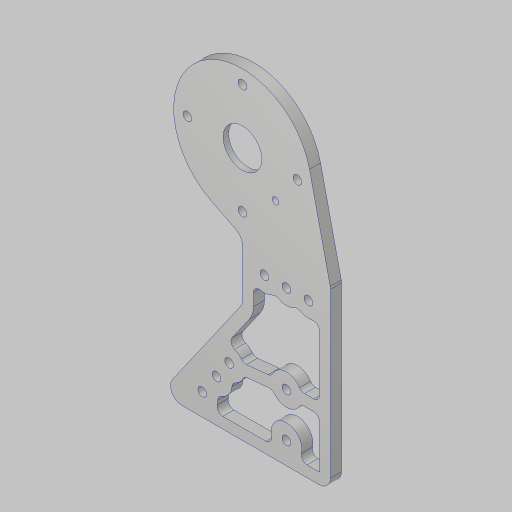
# Autodesk Inventor part: CL7-010
Saved by Autodesk Inventor 2023.5 (Build 275446000, 446)
## iProperties
Created: 2025-03-18
Part Number: CL7-010
Material: Aluminum 6061
Document SubType Name: Modeling
Designer: slick
Density: 2.7 g/cm^3
Appearance: Aluminum - Flat
Author: slick
Autodesk Inventor part; units mm, degrees
ref_plane "YZ Plane" through (0, 0, 0) normal (1, 0, 0) x (0, 1, 0)
ref_plane "XZ Plane" through (0, 0, 0) normal (0, 1, 0) x (-1, 0, 0)
ref_plane "XY Plane" through (0, 0, 0) normal (0, 0, 1) x (1, 0, 0)
sketch "Sketch1" plane through (0, 0, 0) normal (0, 0, 1) x (1, 0, 0)
  line L0 (0, 0) -> (50.8, 0) construction
  line L1 (50.8, 0) -> (50.8, 387.35) construction
  line L2 (50.8, 387.35) -> (0, 387.35) construction
  line L3 (0, 387.35) -> (0, 0) construction
  line L4 (20.8065, 339.141) -> (-226.8638, -14.5688) construction
  line L5 (-226.8638, -14.5688) -> (-247.6703, 0) construction
  line L6 (-247.6703, 0) -> (0, 353.7099) construction
  line L7 (0, 353.7099) -> (20.8065, 339.141) construction
  line L8 (-247.6703, 0) -> (-216.6626, 0) construction
  line L9 (0, 353.7099) -> (0, 309.4263) construction
  dimension "d0" = 50.8
  dimension "d1" = 387.35
  dimension "d2" = 25.4
  dimension "d3" = 431.8
  dimension "d5" = 55
  constraints: 20 end point, 4 parallel, 2 horizontal, 2 perpendicular, 2 point on line, 1 horizontal alignment, 1 vertical, 1 vertical alignment
  measures "d0" distance of L2.end L1.end
  measures "d1" distance of L1.end L0.end
  measures "d2" distance of L4.end L5.end
  measures "d3" distance of L5.end L6.end
  measures "d5" angle of L7 L3
sketch "Sketch2" plane through (0, 0, 0) normal (0, 0, 1) x (1, 0, 0)
  line L0 (0, 0) -> (50.8, 0) construction
  line L1 (50.8, 0) -> (50.8, 387.35) construction
  line L2 (50.8, 387.35) -> (0, 387.35) construction
  line L3 (0, 387.35) -> (0, 0) construction
  line L4 (20.8065, 339.141) -> (-226.8638, -14.5688) construction
  line L5 (-226.8638, -14.5688) -> (-247.6703, 0) construction
  line L6 (-247.6703, 0) -> (0, 353.7099) construction
  line L7 (0, 353.7099) -> (20.8065, 339.141) construction
  line L8 (-247.6703, 0) -> (-216.6626, 0) construction
  line L9 (0, 353.7099) -> (0, 309.4263) construction
  circle A0 centre (0, 431.8) radius 11.176
  circle A1 centre (0, 431.8) radius 23.8125 construction
  circle A2 centre (0, 431.8) radius 39.6875 construction
  line L10 (-47.586, 285.75) -> (0, 353.7099)
  line L11 (0, 387.35) -> (0, 353.7099)
  line L12 (0, 387.35) -> (-17.8729, 396.3647)
  line L13 (50.8, 387.35) -> (50.8, 285.75)
  line L14 (50.8, 285.75) -> (-47.586, 285.75)
  arc A3 (38.7009, 440.5943) -> (-17.8729, 396.3647) centre (0, 431.8) ccw
  line L15 (12.7, 374.65) -> (38.1, 374.65) construction
  line L16 (10.4032, 346.4254) -> (-237.2671, -7.2844) construction
  line L17 (50.8, 387.35) -> (38.7009, 440.5943)
  point P0 (25.4, 0)
  point P1 (-7.667, 320.6184)
  point P2 (-14.9514, 310.2152)
  point P3 (-23.1895, 298.45)
  point P4 (25.4, 374.65)
  point P5 (25.4, 374.65)
  point P6 (25.4, 387.35)
  dimension "d6" = 22.352
  dimension "d7" = 47.625
  dimension "d8" = 15.875
  dimension "d11" = 431.8
  dimension "d12" = 101.6
  dimension "d13" = 25.4
  dimension "d14" = 12.7
  dimension "d15" = 12.7
  dimension "d16" = 14.3627
  dimension "d17" = 12.7
  dimension "d52" = 50.8
  constraints: 16 end point, 5 midpoint, 5 point on line, 4 centre point, 4 point on circle, 3 coincident, 2 perpendicular, 2 tangent, 1 collinear, 1 horizontal, 1 vertical alignment
  measures "d6" diameter of A0
  measures "d7" diameter of A1
  measures "d8" radial gap between concentric circles of A1 A2
  measures "d11" distance from line of L0 A0.centre
  measures "d12" distance between parallel lines of L2 L14
  measures "d13" distance of L15.start L15.end
  measures "d14" distance between parallel lines of L2 L15
  measures "d15" distance of point (-14.951, 310.215) point (-7.667, 320.618)
  measures "d16" distance of point (-14.951, 310.215) point (-23.19, 298.45)
  measures "d17" distance from line of L14 point (-23.19, 298.45)
  measures "d52" distance from line of L1 A0.centre
extrude "Extrusion1" add sketch "Sketch2" along normal blind 6.35
hole "Hole1" at (0, 0, 0) at (50.8, 0, 0) at (-226.8638, -14.5688, 0) at (-247.6703, 0, 0) at (-216.6626, 0, 0) at (-7.667, 320.6184, 0) at (-14.9514, 310.2152, 0) at (-23.1895, 298.45, 0) at (12.7, 374.65, 0) at (25.4, 374.65, 0) at (38.1, 374.65, 0) direction (0, 0, 1) diameter 5.1054 end through all clearance for "Flat Head Machine Screw (82)" size "#10" standard "Ansi Unified Screw Threads"
fillet "Fillet1" radius 6.604 5 edges at (0, 353.7099, 3.175) (-47.586, 285.75, 3.175) (50.8, 285.75, 3.175) (0, 387.35, 3.175) (50.8, 387.35, 3.175)
sketch "Sketch3" plane through (0, 0, 0) normal (0, 0, -1) x (-1, 0, 0)
  arc A0 (-50.8, 292.354) -> (-44.196, 285.75) centre (-44.196, 292.354) ccw construction
  line L0 (34.8998, 285.75) -> (-44.196, 285.75) construction
  arc A1 (34.8998, 285.75) -> (40.3095, 296.1419) centre (34.8998, 292.354) ccw construction
  line L1 (1.1943, 352.0042) -> (40.3095, 296.1419) construction
  arc A2 (0, 355.7921) -> (1.1943, 352.0042) centre (6.604, 355.7921) ccw construction
  line L2 (0, 383.2845) -> (0, 355.7921) construction
  line L3 (17.8729, 396.3647) -> (3.63, 389.1809) construction
  arc A3 (17.8729, 396.3647) -> (-38.7009, 440.5943) centre (0, 431.8) ccw construction
  line L4 (-50.8, 292.354) -> (-50.8, 386.6091) construction
  circle A4 centre (-25.4, 374.65) radius 2.5527 construction
  circle A5 centre (23.1895, 298.45) radius 2.5527 construction
  circle A6 centre (7.667, 320.6184) radius 2.5527 construction
  circle A7 centre (14.9514, 310.2152) radius 2.5527 construction
  circle A8 centre (-12.7, 374.65) radius 2.5527 construction
  circle A9 centre (-38.1, 374.65) radius 2.5527 construction
  circle A10 centre (0, 431.8) radius 11.176 construction
  circle A11 centre (0, 431.8) radius 23.8125
  circle A12 centre (0, 431.8) radius 11.176 construction
  circle A13 centre (0, 431.8) radius 31.75 construction
  line L5 (-50.6358, 388.0725) -> (-38.7009, 440.5943) projected
  arc A14 (-50.6358, 388.0725) -> (-50.8, 386.6091) centre (-44.196, 386.6091) ccw projected
  arc A15 (3.63, 389.1809) -> (0, 383.2845) centre (6.604, 383.2845) ccw projected
  point P0 (0, 0)
  point P1 (0, 463.55)
  point P2 (-31.75, 431.8)
  point P3 (0, 400.05)
  point P4 (31.75, 431.8)
  dimension "d29" = 63.5
  dimension "d28" = 47.625
  dimension "d32" = 360
  constraints: 2 coincident, 2 vertical alignment, 1 centre point, 7 other
  measures "d28" diameter of A11
extrude "Extrusion2" cut sketch "Sketch3" against normal blind 3.175
hole "Hole2" at (0, 463.55, 0) at (31.75, 431.8, 0) at (0, 400.05, 0) at (-31.75, 431.8, 0) direction (0, 0, 1) diameter 5.1054 end through all clearance for "Flat Head Machine Screw (82)" size "#10" standard "Ansi Unified Screw Threads"
sketch "Sketch4" plane through (0, 0, 6.35) normal (0, 0, 1) x (1, 0, 0)
  line L0 (0, 0) -> (50.8, 0) construction
  line L1 (-34.8998, 285.75) -> (44.196, 285.75) construction
  point P0 (25.4, 323.85)
  point P1 (25.4, 298.45)
  point P2 (25.4, 0)
  dimension "d43" = 25.4
  dimension "d44" = 12.7
  constraints: 2 vertical alignment, 1 midpoint
  measures "d43" distance of point (25.4, 323.85) point (25.4, 298.45)
  measures "d44" distance from line of L1 point (25.4, 298.45)
hole "Hole3" at (25.4, 323.85, 6.35) at (25.4, 298.45, 6.35) direction (0, 0, -1) diameter 5.1054 end through all clearance for "Flat Head Machine Screw (82)" size "#10" standard "Ansi Unified Screw Threads"
sketch "Sketch5" plane through (0, 0, 6.35) normal (0, 0, 1) x (1, 0, 0)
  circle A0 centre (25.4, 323.85) radius 2.5527 construction
  circle A1 centre (25.4, 298.45) radius 2.5527 construction
  circle A2 centre (0, 400.05) radius 2.5527 construction
  circle A3 centre (0, 463.55) radius 2.5527 construction
  circle A4 centre (31.75, 431.8) radius 2.5527 construction
  circle A5 centre (-31.75, 431.8) radius 2.5527 construction
  circle A6 centre (0, 431.8) radius 11.176 construction
  arc A7 (50.8, 386.6091) -> (50.6358, 388.0725) centre (44.196, 386.6091) ccw construction
  line L0 (50.6358, 388.0725) -> (38.7009, 440.5943) construction
  arc A8 (38.7009, 440.5943) -> (-17.8729, 396.3647) centre (0, 431.8) ccw construction
  line L1 (-17.8729, 396.3647) -> (-3.63, 389.1809) construction
  arc A9 (0, 383.2845) -> (-3.63, 389.1809) centre (-6.604, 383.2845) ccw construction
  line L2 (0, 383.2845) -> (0, 355.7921) construction
  arc A10 (-1.1943, 352.0042) -> (0, 355.7921) centre (-6.604, 355.7921) ccw construction
  line L3 (-1.1943, 352.0042) -> (-40.3095, 296.1419) construction
  arc A11 (-40.3095, 296.1419) -> (-34.8998, 285.75) centre (-34.8998, 292.354) ccw construction
  line L4 (-34.8998, 285.75) -> (44.196, 285.75) construction
  arc A12 (44.196, 285.75) -> (50.8, 292.354) centre (44.196, 292.354) ccw construction
  line L5 (50.8, 292.354) -> (50.8, 386.6091) construction
  circle A13 centre (38.1, 374.65) radius 2.5527 construction
  circle A14 centre (12.7, 374.65) radius 2.5527 construction
  circle A15 centre (-14.9514, 310.2152) radius 2.5527 construction
  circle A16 centre (-7.667, 320.6184) radius 2.5527 construction
  circle A17 centre (-23.1895, 298.45) radius 2.5527 construction
  circle A18 centre (25.4, 374.65) radius 2.5527 construction
  line L6 (6.35, 355.7921) -> (6.35, 383.2845) construction
  arc A19 (6.35, 383.2845) -> (-0.7703, 394.8505) centre (-6.604, 383.2845) ccw construction
  line L7 (-0.7703, 394.8505) -> (-15.0132, 402.0344) construction
  arc A20 (32.5087, 439.1872) -> (-15.0132, 402.0344) centre (0, 431.8) ccw construction
  line L8 (32.5087, 439.1872) -> (44.4437, 386.6654) construction
  arc A21 (44.45, 386.6091) -> (44.4437, 386.6654) centre (44.196, 386.6091) ccw construction
  line L9 (44.45, 386.6091) -> (44.45, 292.354) construction
  arc A22 (44.196, 292.1) -> (44.45, 292.354) centre (44.196, 292.354) ccw construction
  line L10 (44.196, 292.1) -> (-34.8998, 292.1) construction
  arc A23 (-35.1079, 292.4997) -> (-34.8998, 292.1) centre (-34.8998, 292.354) ccw construction
  line L11 (-35.1079, 292.4997) -> (4.0073, 348.362) construction
  arc A24 (4.0073, 348.362) -> (6.35, 355.7921) centre (-6.604, 355.7921) ccw construction
  circle A25 centre (25.4, 323.85) radius 8.9027 construction
  circle A26 centre (12.7, 374.65) radius 8.9027 construction
  circle A27 centre (25.4, 374.65) radius 8.9027 construction
  circle A28 centre (38.1, 374.65) radius 8.9027 construction
  circle A29 centre (-7.667, 320.6184) radius 2.5527 construction
  circle A30 centre (-7.667, 320.6184) radius 8.9027 construction
  line L12 (-7.667, 320.6184) -> (25.4, 323.85) construction
  line L13 (25.4, 323.85) -> (44.45, 323.85) construction
  arc A31 (6.35, 368.4102) -> (19.05, 368.4102) centre (12.7, 374.65) ccw
  arc A32 (19.05, 368.4102) -> (31.75, 368.4102) centre (25.4, 374.65) ccw
  arc A33 (31.75, 368.4102) -> (44.45, 368.4102) centre (38.1, 374.65) ccw
  arc A34 (-1.1943, 352.0042) -> (0, 355.7921) centre (-6.604, 355.7921) ccw construction
  arc A35 (4.0073, 348.362) -> (6.35, 355.7921) centre (-6.604, 355.7921) ccw
  line L14 (6.35, 368.4102) -> (6.35, 355.7921)
  line L15 (44.45, 323.85) -> (44.45, 368.4102)
  line L16 (4.0073, 348.362) -> (-9.2896, 329.372)
  circle A36 centre (0, 431.8) radius 33.3375 construction
  circle A37 centre (0, 400.05) radius 8.9027 construction
  circle A38 centre (31.75, 431.8) radius 2.5527 construction
  circle A39 centre (31.75, 431.8) radius 8.9027 construction
  circle A40 centre (0, 431.8) radius 36.5125 construction
  arc A41 (8.0168, 396.1785) -> (35.6215, 423.7832) centre (0, 431.8) ccw
  arc A42 (3.2058, 391.7445) -> (8.0168, 396.1785) centre (0, 400.05) ccw
  arc A43 (35.6215, 423.7832) -> (35.9688, 423.9604) centre (31.75, 431.8) ccw
  arc A44 (44.45, 386.6091) -> (44.4437, 386.6654) centre (44.196, 386.6091) ccw
  arc A45 (6.35, 383.2845) -> (3.2058, 391.7445) centre (-6.604, 383.2845) ccw
  arc A46 (19.05, 380.8898) -> (6.35, 380.8898) centre (12.7, 374.65) ccw
  arc A47 (31.75, 380.8898) -> (19.05, 380.8898) centre (25.4, 374.65) ccw
  arc A48 (44.45, 380.8898) -> (31.75, 380.8898) centre (38.1, 374.65) ccw
  line L17 (6.35, 383.2845) -> (6.35, 380.8898)
  line L18 (44.45, 380.8898) -> (44.45, 386.6091)
  line L19 (44.4437, 386.6654) -> (35.9688, 423.9604)
  circle A49 centre (-23.1895, 298.45) radius 8.9027 construction
  circle A50 centre (25.4, 298.45) radius 8.9027 construction
  circle A51 centre (-14.9514, 310.2152) radius 8.9027 construction
  line L20 (-7.9758, 323.7784) -> (25.2452, 327.025) construction
  line L21 (25.2452, 327.025) -> (44.45, 327.025) construction
  line L22 (-7.3582, 317.4585) -> (25.5548, 320.675) construction
  line L23 (25.5548, 320.675) -> (44.45, 320.675) construction
  line L24 (0.302, 324.5874) -> (16.8133, 326.201)
  line L25 (33.7173, 327.025) -> (44.45, 327.025)
  line L26 (44.45, 320.675) -> (33.7173, 320.675)
  line L27 (17.431, 319.8811) -> (0.9197, 318.2675)
  line L28 (44.45, 320.675) -> (44.45, 292.354)
  line L29 (44.196, 292.1) -> (31.6398, 292.1)
  line L30 (19.1602, 292.1) -> (-16.9497, 292.1)
  arc A52 (-16.9497, 292.1) -> (-14.7603, 301.3146) centre (-23.1895, 298.45) ccw
  arc A53 (-14.7603, 301.3146) -> (-6.1979, 311.8378) centre (-14.9514, 310.2152) ccw
  arc A54 (-6.1979, 311.8378) -> (0.9197, 318.2675) centre (-7.667, 320.6184) ccw
  arc A55 (17.431, 319.8811) -> (33.7173, 320.675) centre (25.4, 323.85) ccw
  arc A56 (33.7173, 327.025) -> (16.8133, 326.201) centre (25.4, 323.85) ccw
  arc A57 (31.6398, 292.1) -> (19.1602, 292.1) centre (25.4, 298.45) ccw
  arc A58 (44.196, 292.1) -> (44.45, 292.354) centre (44.196, 292.354) ccw
  arc A59 (0.302, 324.5874) -> (-9.2896, 329.372) centre (-7.667, 320.6184) ccw
  point P0 (0, 0)
  point P1 (1.1935, 321.4844)
  point P2 (34.3027, 323.85)
  point P3 (16.5395, 322.9841)
  point P4 (44.45, 386.6091)
  dimension "d53" = 6.35
  dimension "d54" = 6.35
  dimension "d55" = 3.175
  dimension "d60" = 3.175
  dimension "d61" = 3.175
  constraints: 88 point on circle, 50 end point, 38 centre point, 30 coincident, 21 point on line, 11 equal radius, 4 collinear, 1 perpendicular, 13 other
  measures "d53" distance between parallel lines of L2 L6
  measures "d54" radial gap between concentric circles of A0 A25
  measures "d55" radial gap between concentric circles of A36 A40
  measures "d60" distance between parallel lines of L12 L20
  measures "d61" distance between parallel lines of L12 L22
extrude "Extrusion3" cut sketch "Sketch5" against normal through all contours A31 A32 A33 L15 L25 A56 L24 A59 L16 A35 L14 | L28 A58 L29 A57 L30 A52 A53 A54 L27 A55 L26
fillet "Fillet2" radius 3.302 18 edges at (-16.9497, 292.1, 3.175) (19.1602, 292.1, 3.175) (31.6398, 292.1, 3.175) (44.45, 320.675, 3.175) (33.7173, 320.675, 3.175) (17.431, 319.8811, 3.175) (0.9197, 318.2675, 3.175) (-6.1979, 311.8378, 3.175) (-14.7603, 301.3146, 3.175) (16.8133, 326.201, 3.175) (33.7173, 327.025, 3.175) (44.45, 327.025, 3.175) (44.45, 368.4102, 3.175) (31.75, 368.4102, 3.175) (19.05, 368.4102, 3.175) (6.35, 368.4102, 3.175) (-9.2896, 329.372, 3.175) (0.302, 324.5874, 3.175)
sketch "Sketch6" plane through (0, 0, 6.35) normal (0, 0, 1) x (1, 0, 0)
  line L0 (35.7442, 320.675) -> (41.148, 320.675) construction
  arc A0 (44.45, 317.373) -> (41.148, 320.675) centre (41.148, 317.373) ccw construction
  line L1 (44.45, 317.373) -> (44.45, 292.354) construction
  arc A1 (44.196, 292.1) -> (44.45, 292.354) centre (44.196, 292.354) ccw construction
  line L2 (44.196, 292.1) -> (37.218, 292.1) construction
  arc A2 (34.0206, 296.2266) -> (37.218, 292.1) centre (37.218, 295.402) ccw construction
  arc A3 (34.0206, 296.2266) -> (16.7794, 296.2266) centre (25.4, 298.45) ccw construction
  arc A4 (13.582, 292.1) -> (16.7794, 296.2266) centre (13.582, 295.402) ccw construction
  line L3 (13.582, 292.1) -> (-11.3716, 292.1) construction
  arc A5 (-14.5689, 296.2266) -> (-11.3716, 292.1) centre (-11.3716, 295.402) ccw construction
  arc A6 (-14.5689, 296.2266) -> (-14.2883, 298.6122) centre (-23.1895, 298.45) ccw construction
  arc A7 (-12.0595, 301.7953) -> (-14.2883, 298.6122) centre (-10.9869, 298.6724) ccw construction
  arc A8 (-12.0595, 301.7953) -> (-6.0668, 309.6487) centre (-14.9514, 310.2152) ccw construction
  arc A9 (-4.096, 312.4633) -> (-6.0668, 309.6487) centre (-2.7715, 309.4386) ccw construction
  arc A10 (-4.096, 312.4633) -> (0.3023, 316.6501) centre (-7.667, 320.6184) ccw construction
  arc A11 (2.937, 318.4646) -> (0.3023, 316.6501) centre (3.2581, 315.1783) ccw construction
  line L4 (2.937, 318.4646) -> (15.4136, 319.6839) construction
  arc A12 (18.3497, 318.4138) -> (15.4136, 319.6839) centre (15.7348, 316.3976) ccw construction
  arc A13 (18.3497, 318.4138) -> (32.9456, 319.1254) centre (25.4, 323.85) ccw construction
  arc A14 (35.7442, 320.675) -> (32.9456, 319.1254) centre (35.7442, 317.373) ccw construction
  arc A15 (10.4766, 366.0294) -> (17.332, 367.0472) centre (12.7, 374.65) ccw construction
  arc A16 (20.768, 367.0472) -> (17.332, 367.0472) centre (19.05, 364.2273) ccw construction
  arc A17 (20.768, 367.0472) -> (30.032, 367.0472) centre (25.4, 374.65) ccw construction
  arc A18 (33.468, 367.0472) -> (30.032, 367.0472) centre (31.75, 364.2273) ccw construction
  arc A19 (33.468, 367.0472) -> (40.3234, 366.0294) centre (38.1, 374.65) ccw construction
  arc A20 (44.45, 362.832) -> (40.3234, 366.0294) centre (41.148, 362.832) ccw construction
  line L5 (44.45, 362.832) -> (44.45, 330.327) construction
  arc A21 (41.148, 327.025) -> (44.45, 330.327) centre (41.148, 330.327) ccw construction
  line L6 (41.148, 327.025) -> (35.7442, 327.025) construction
  arc A22 (32.9456, 328.5746) -> (35.7442, 327.025) centre (35.7442, 330.327) ccw construction
  arc A23 (32.9456, 328.5746) -> (17.4307, 327.8183) centre (25.4, 323.85) ccw construction
  arc A24 (14.796, 326.0038) -> (17.4307, 327.8183) centre (14.4748, 329.2902) ccw construction
  line L7 (14.796, 326.0038) -> (2.3194, 324.7845) construction
  arc A25 (-0.6167, 326.0546) -> (2.3194, 324.7845) centre (1.9982, 328.0709) ccw construction
  arc A26 (-0.6167, 326.0546) -> (-4.5437, 328.9553) centre (-7.667, 320.6184) ccw construction
  arc A27 (-6.0901, 333.9414) -> (-4.5437, 328.9553) centre (-3.3853, 332.0474) ccw construction
  line L8 (-6.0901, 333.9414) -> (4.0073, 348.362) construction
  arc A28 (4.0073, 348.362) -> (6.35, 355.7921) centre (-6.604, 355.7921) ccw construction
  line L9 (6.35, 355.7921) -> (6.35, 362.832) construction
  arc A29 (10.4766, 366.0294) -> (6.35, 362.832) centre (9.652, 362.832) ccw construction
  circle A30 centre (25.4, 323.85) radius 2.5527 construction
  circle A31 centre (25.4, 298.45) radius 2.5527 construction
  circle A32 centre (0, 400.05) radius 2.5527 construction
  circle A33 centre (0, 463.55) radius 2.5527 construction
  circle A34 centre (31.75, 431.8) radius 2.5527 construction
  circle A35 centre (-31.75, 431.8) radius 2.5527 construction
  circle A36 centre (0, 431.8) radius 11.176 construction
  arc A37 (50.8, 386.6091) -> (50.6358, 388.0725) centre (44.196, 386.6091) ccw construction
  line L10 (50.6358, 388.0725) -> (38.7009, 440.5943) construction
  arc A38 (38.7009, 440.5943) -> (-17.8729, 396.3647) centre (0, 431.8) ccw construction
  line L11 (-17.8729, 396.3647) -> (-3.63, 389.1809) construction
  arc A39 (0, 383.2845) -> (-3.63, 389.1809) centre (-6.604, 383.2845) ccw construction
  line L12 (0, 383.2845) -> (0, 355.7921) construction
  arc A40 (-1.1943, 352.0042) -> (0, 355.7921) centre (-6.604, 355.7921) ccw construction
  line L13 (-1.1943, 352.0042) -> (-40.3095, 296.1419) construction
  arc A41 (-40.3095, 296.1419) -> (-34.8998, 285.75) centre (-34.8998, 292.354) ccw construction
  line L14 (-34.8998, 285.75) -> (44.196, 285.75) construction
  arc A42 (44.196, 285.75) -> (50.8, 292.354) centre (44.196, 292.354) ccw construction
  line L15 (50.8, 292.354) -> (50.8, 386.6091) construction
  circle A43 centre (38.1, 374.65) radius 2.5527 construction
  circle A44 centre (12.7, 374.65) radius 2.5527 construction
  circle A45 centre (-14.9514, 310.2152) radius 2.5527 construction
  circle A46 centre (-7.667, 320.6184) radius 2.5527 construction
  circle A47 centre (-23.1895, 298.45) radius 2.5527 construction
  circle A48 centre (25.4, 374.65) radius 2.5527 construction
  point P0 (0, 0)
  point P1 (19.05, 414.9995)
  dimension "d63" = 25.4
  dimension "d64" = 19.05
  measures "d63" distance of point (19.05, 414.999) A36.centre
  measures "d64" distance from line of point (19.05, 414.999) L12
hole "Hole4" at (19.05, 414.9995, 6.35) direction (0, 0, -1) diameter 3.9624 end through all thread size "10-32 UNF" class "2B" standard "ANSI Unified Screw Threads"
body "Solid1"
